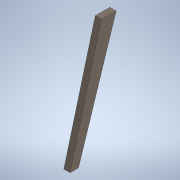
# Autodesk Inventor part: Leg
Saved by Autodesk Inventor 2022 (Build 260153000, 153)
## iProperties
Created: 2022-01-15
Part Number: Leg
Material: Generic
Document SubType Name: Modeling
Designer: dangl
Density: 1 g/cm^3
Appearance: Default
Author: dangl
Autodesk Inventor part; units mm, degrees
ref_plane "YZ Plane" through (0, 0, 0) normal (1, 0, 0) x (0, 1, 0)
ref_plane "XZ Plane" through (0, 0, 0) normal (0, 1, 0) x (-1, 0, 0)
ref_plane "XY Plane" through (0, 0, 0) normal (0, 0, 1) x (1, 0, 0)
sketch "Sketch1" plane through (0, 0, 0) normal (1, 0, 0) x (0, 1, 0)
  line L0 (-19.05, 429.9938) -> (-19.05, -429.9938) projected
  line L1 (-19.05, 312.394) -> (-730.25, 502.9594)
  line L2 (-730.25, 502.9594) -> (-730.25, 452.1594)
  line L3 (-730.25, 452.1594) -> (-19.05, 223.494)
  line L4 (-19.05, 312.394) -> (-19.05, 223.494)
  point P0 (0, 0)
  dimension "d0" = 88.9
  dimension "d1" = 50.8
  dimension "d2" = 711.2
  dimension "d3" = 75
  constraints: 8 end point, 2 point on line, 1 collinear, 1 vertical
  measures "d0" distance of L3.end L1.start
  measures "d1" distance of L1.end L2.end
  measures "d2" distance between parallel lines of L2 L0
  measures "d3" angle of L0 L1
extrude "Extrusion1" add sketch "Sketch1" along normal mid plane 38.1
body "Solid1"
